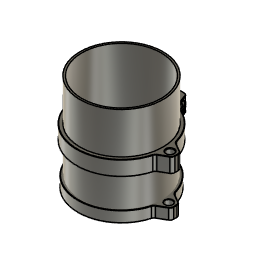
rear_44mm_dia (Autodesk Fusion 360 design; units mm, degrees)
Autodesk Fusion 360 part; units mm, degrees
sketch "Sketch1" plane through (0, 0, 0) normal (0, 0, 1) x (1, 0, 0)
  circle A0 centre (0, 0) radius 22.2
  circle A1 centre (0, 0) radius 21.2
  dimension "d1" = 44.4
  dimension "d2" = 1
  constraint coincident A0.centre A1.centre
  measures "d1" diameter of A0
  measures "d2" distance of A0 A1
extrude "Extrude1" add sketch "Sketch1" along normal blind 50 makes body 1
ref_plane "WorkPlane1" through (0, 0, 20) normal (0, 0, 1) x (1, 0, 0)
sketch "Sketch2" plane through (0, 0, 20) normal (0, 0, 1) x (1, 0, 0)
  circle A0 centre (0, 0) radius 22
  circle A1 centre (0, 0) radius 24
  line L0 (0, 0) -> (0, 24) construction
  line L1 (-6.9118, 22.9832) -> (-4, 30.9832)
  line L2 (-4, 30.9832) -> (0, 30.9832)
  line L3 (0, 30.9832) -> (0, 24)
  line L4 (-6.9118, 22.9832) -> (0, 22.9832) construction
  line L5 (-4, 30.9832) -> (-4, 22.9832) construction
  line L6 (0, 0) -> (-0.3072, 21.9979)
  line L7 (-0.3072, 21.9979) -> (-0.3072, 30.9832)
  line L8 (6.9118, 22.9832) -> (4, 30.9832)
  line L9 (4, 30.9832) -> (0, 30.9832)
  line L10 (0.3072, 21.9979) -> (0.3072, 30.9832)
  line L11 (0, 0) -> (0.3072, 21.9979)
  circle A2 centre (-26, 0) radius 2
  line L12 (0, 0) -> (-24, 0) construction
  line L13 (-23.3435, 5.5752) -> (-29.5, 2.0207)
  line L14 (-29.5, 2.0207) -> (-29.5, 0)
  line L15 (-23.3435, -5.5752) -> (-29.5, -2.0207)
  line L16 (-29.5, -2.0207) -> (-29.5, 0)
  line L17 (23.3435, 5.5752) -> (29.5, 2.0207)
  line L18 (29.5, 2.0207) -> (29.5, 0)
  line L19 (29.5, -2.0207) -> (29.5, 0)
  line L20 (23.3435, -5.5752) -> (29.5, -2.0207)
  circle A3 centre (26, 0) radius 2
  dimension "d6" = 44
  dimension "d7" = 2
  dimension "d8" = 8
  dimension "d9" = 20
  dimension "d10" = 4
  dimension "d11" = 0.8
  dimension "d14" = 4
  dimension "d16" = 3.5
  dimension "d17" = 3.5
  dimension "d18" = 120
  constraint coincident A0.centre A1.centre
  constraint coincident A1 L0.end
  constraint vertical L0
  constraint coincident A1 L1.start
  constraint horizontal L2
  constraint perpendicular L2 L3
  constraint coincident L0 L4.end
  constraint horizontal L4
  constraint coincident L4 L5.end
  constraint perpendicular L4 L5
  constraint coincident A0 L6.end
  constraint coincident L2 L7.end
  constraint perpendicular L2 L7
  constraint symmetric L0 L1.start L8.start
  constraint symmetric L0 L1.end L8.end
  constraint symmetric L0 L2.end L3.start
  constraint symmetric L0 A0.centre A1.centre
  constraint symmetric L0 L6.end L10.start
  constraint symmetric L0 L7.end L10.end
  constraint coincident A1 L12.end
  constraint horizontal L12
  constraint coincident A2.centre L12
  constraint coincident A1 L13.start
  constraint vertical L14
  constraint tangent A1 A2
  constraint coincident L12 L14.end
  constraint symmetric L12 L13.start L15.start
  constraint symmetric L12 L13.end L15.end
  constraint symmetric L12 L14.end L16.end
  constraint symmetric L0 A2 A3
  constraint symmetric L0 L13.start L17.start
  constraint symmetric L0 L13.end L17.end
  constraint symmetric L0 L14.end L18.end
  constraint symmetric L0 L15.start L20.start
  constraint symmetric L0 L15.end L19.start
  measures "d6" diameter of A0
  measures "d7" distance of A0 A1
  measures "d8" distance of L2 L4
  measures "d9" angle of L1 L5
  measures "d10" distance of L1.end L3
  measures "d11" angle of L0 L6
  measures "d14" diameter of A2
  measures "d16" distance of A2.centre L14
  measures "d17" distance of A2.centre L13
  measures "d18" angle of L13 L14
extrude "Extrude2" add sketch "Sketch2" along normal blind 8 separate body contours A0 A1 L7 L10 | A1 L8 L9 L10 | A1 L1 L2 L7 | A1 L17 L18 L19 L20 | A1 L13 L14 L15 L16 picked at (22.5633, -1.6974) makes body 2
sketch "Sketch3" plane through (-0.3072, 0, 0) normal (1, 0, 0) x (0, 1, 0)
  line L0 (21.9979, 20) -> (30.9832, 20)
  line L1 (30.9832, 20) -> (30.9832, 28)
  line L2 (30.9832, 28) -> (21.9979, 28)
  line L3 (21.9979, 28) -> (21.9979, 20)
  line L4 (21.9979, 24) -> (30.9832, 24) construction
  line L5 (26.4905, 28) -> (26.4905, 20) construction
  circle A0 centre (26.9832, 24) radius 1.4
  dimension "d19" = 2.8
  dimension "d20" = 4
  constraint midpoint L3 L4.start
  constraint midpoint L1 L4.end
  constraint midpoint L2 L5.start
  constraint perpendicular L2 L5
  constraint coincident L4 A0.centre
  measures "d19" diameter of A0
  measures "d20" distance of L1 A0.centre
extrude "Extrude3" cut sketch "Sketch3" along normal through all and the other way through all contours A0 bodies 2
sketch "Sketch4" plane through (0, 0, 28) normal (0, 0, 1) x (-1, 0, 0)
  circle A0 centre (-26, 0) radius 2
  circle A1 centre (26, 0) radius 2
  arc A2 (23.3435, 5.5752) -> (-23.3435, 5.5752) centre (0, 0) ccw
  line L0 (-23.3435, 5.5752) -> (-29.5, 2.0207)
  line L1 (-29.5, 2.0207) -> (-29.5, -2.0207)
  line L2 (-29.5, -2.0207) -> (-23.3435, -5.5752)
  arc A3 (-23.3435, -5.5752) -> (-6.9118, -22.9832) centre (0, 0) ccw
  line L3 (-6.9118, -22.9832) -> (-4, -30.9832)
  line L4 (-4, -30.9832) -> (-0.3072, -30.9832)
  line L5 (-0.3072, -30.9832) -> (-0.3072, -21.9979)
  arc A4 (0.3072, -21.9979) -> (-0.3072, -21.9979) centre (0, 0) ccw
  line L6 (0.3072, -21.9979) -> (0.3072, -30.9832)
  line L7 (0.3072, -30.9832) -> (4, -30.9832)
  line L8 (4, -30.9832) -> (6.9118, -22.9832)
  arc A5 (6.9118, -22.9832) -> (23.3435, -5.5752) centre (0, 0) ccw
  line L9 (23.3435, -5.5752) -> (29.5, -2.0207)
  line L10 (29.5, -2.0207) -> (29.5, 2.0207)
  line L11 (29.5, 2.0207) -> (23.3435, 5.5752)
  line L12 (-4, -30.9832) -> (-4, -21.6333) construction
  constraint coincident L3.end L4.start
  constraint coincident A4 L12.end
  constraint perpendicular L4 L12
sketch "Sketch5" plane through (0, 0, 20) normal (0, 0, -1) x (1, 0, 0)
  circle A0 centre (26, 0) radius 2
  circle A1 centre (-26, 0) radius 2
  arc A2 (23.3435, 5.5752) -> (-23.3435, 5.5752) centre (0, 0) ccw
  line L0 (-23.3435, 5.5752) -> (-29.5, 2.0207)
  line L1 (-29.5, 2.0207) -> (-29.5, -2.0207)
  line L2 (-29.5, -2.0207) -> (-23.3435, -5.5752)
  arc A3 (-23.3435, -5.5752) -> (-6.9118, -22.9832) centre (0, 0) ccw
  line L3 (-6.9118, -22.9832) -> (-4, -30.9832)
  line L4 (-4, -30.9832) -> (-0.3072, -30.9832)
  line L5 (-0.3072, -30.9832) -> (-0.3072, -21.9979)
  arc A4 (0.3072, -21.9979) -> (-0.3072, -21.9979) centre (0, 0) ccw
  line L6 (0.3072, -21.9979) -> (0.3072, -30.9832)
  line L7 (0.3072, -30.9832) -> (4, -30.9832)
  line L8 (4, -30.9832) -> (6.9118, -22.9832)
  arc A5 (6.9118, -22.9832) -> (23.3435, -5.5752) centre (0, 0) ccw
  line L9 (23.3435, -5.5752) -> (29.5, -2.0207)
  line L10 (29.5, -2.0207) -> (29.5, 2.0207)
  line L11 (29.5, 2.0207) -> (23.3435, 5.5752)
  line L12 (4, -30.9832) -> (4, -21.6333) construction
ref_plane "WorkPlane2" through (4, 30.9832, 28) normal (-1, 0, 0) x (0, -1, 0)
sketch "Sketch6" plane through (4, 0, 0) normal (-1, 0, 0) x (0, -1, 0)
  circle A0 centre (-26.9832, 24) radius 1.4
  circle A1 centre (-26.9832, 24) radius 1.4
  circle A2 centre (-26.9832, 24) radius 3
  dimension "d23" = 6
  constraint concentric A0 A2
  measures "d23" diameter of A2
extrude "Extrude4" cut sketch "Sketch6" against normal through all bodies 2
sketch "Sketch7" plane through (0.3072, 0, 0) normal (-1, 0, 0) x (0, -1, 0)
  circle A0 centre (-26.9832, 24) radius 1.4
  line L0 (-30.9832, 20) -> (-21.9979, 20)
  line L1 (-21.9979, 20) -> (-21.9979, 28)
  line L2 (-21.9979, 28) -> (-30.9832, 28)
  line L3 (-30.9832, 28) -> (-30.9832, 20)
  circle A1 centre (-26.9832, 24) radius 1.7
  dimension "d28" = 3.4
  constraint concentric A0 A1
  measures "d28" diameter of A1
extrude "Extrude6" cut sketch "Sketch7" against normal up to surface (3.6928 mm away) contours A1 bodies 2
fillet "Fillet1" radius 2 12 edges at (-29.5, -2.0207, 24) (-23.3435, -5.5752, 24) (-29.5, 2.0207, 24) (-23.3435, 5.5752, 24) (23.3435, -5.5752, 24) (29.5, -2.0207, 24) (29.5, 2.0207, 24) (23.3435, 5.5752, 24) (6.9118, 22.9832, 24) (-6.9118, 22.9832, 24) (4, 30.9832, 24) (-4, 30.9832, 24) on bodies 2
fillet "Fillet2" radius 0.5 4 edges at (0.3072, 30.9832, 24) (-0.3072, 30.9832, 24) (0.3072, 21.9979, 24) (-0.3072, 21.9979, 24) on bodies 2
chamfer "Chamfer1" distance 0.2 angle 45 4 edges at (4, 28.5682, 23.3853) (0.3072, 28.5682, 24.6147) (-0.3072, 25.6779, 24.5063) (-5.9654, 25.5832, 24) on bodies 2
fillet "Fillet5" radius 0.2 3 edges at (4, 29.7802, 22.9152) (6.5478, 23.9832, 24) (4.3316, 29.9832, 24) on bodies 2
chamfer "Chamfer2" distance 0.2 angle 45 32 edges at (-23.4884, 5.6646, 28) (-17.4982, 16.4259, 28) (-7.0551, 23.1595, 28) (-5.5281, 26.7847, 28) (-3.7467, 30.6215, 28) (-1.7034, 30.9832, 28) (-0.4536, 30.8368, 28) (-0.3072, 26.4844, 28) (-0.4473, 22.1384, 28) (0, -22, 28) (0.4473, 22.1384, 28) (0.3072, 26.4844, 28) (0.4536, 30.8368, 28) (1.7034, 30.9832, 28) (3.7467, 30.6215, 28) (5.5281, 26.7847, 28) (7.0551, 23.1595, 28) (17.4982, 16.4259, 28) (23.4884, 5.6646, 28) (26.2856, 3.8765, 28) (29.2321, 1.866, 28) (29.5, 0, 28) (29.2321, -1.866, 28) (26.2856, -3.8765, 28) (23.4884, -5.6646, 28) (0, -24, 28) (-23.4884, -5.6646, 28) (-26.2856, -3.8765, 28) (-29.2321, -1.866, 28) (-29.5, 0, 28) (-29.2321, 1.866, 28) (-26.2856, 3.8765, 28) on bodies 2
chamfer "Chamfer3" distance 0.3 angle 45 35 edges at (-27.8647, 0.7232, 28) (24.1353, 0.7232, 28) (26.2856, 3.8765, 20) (29.2321, 1.866, 20) (29.5, 0, 20) (29.2321, -1.866, 20) (26.2856, -3.8765, 20) (23.4884, -5.6646, 20) (0, -24, 20) (-23.4884, -5.6646, 20) (-26.2856, -3.8765, 20) (-29.2321, -1.866, 20) (-29.5, 0, 20) (-29.2321, 1.866, 20) (-26.2856, 3.8765, 20) (-23.4884, 5.6646, 20) (-17.4982, 16.4259, 20) (-7.0551, 23.1595, 20) (-5.5281, 26.7847, 20) (-3.7467, 30.6215, 20) (-1.7034, 30.9832, 20) (-0.4536, 30.8368, 20) (-0.3072, 26.4844, 20) (-0.4473, 22.1384, 20) (0, -22, 20) (0.4473, 22.1384, 20) (0.3072, 26.4844, 20) (0.4536, 30.8368, 20) (1.7034, 30.9832, 20) (3.7467, 30.6215, 20) (5.5281, 26.7847, 20) (7.0551, 23.1595, 20) (17.4982, 16.4259, 20) (23.4884, 5.6646, 20) (24.1353, 0.7232, 20) on bodies 2
sketch "Sketch8" plane through (0, 0, 0) normal (0, 0, 1) x (1, 0, 0)
  circle A0 centre (0, 0) radius 21.3
  circle A1 centre (0, 0) radius 23.3
  line L0 (22.6198, 5.5889) -> (28.8, 2.0207)
  line L1 (28.8, 2.0207) -> (28.8, 0)
  line L2 (0, 0) -> (23.3, 0) construction
  line L3 (22.6198, -5.5889) -> (28.8, -2.0207)
  line L4 (28.8, -2.0207) -> (28.8, 0)
  line L5 (0, 0) -> (0, 21.3) construction
  line L6 (-22.6198, 5.5889) -> (-28.8, 2.0207)
  line L7 (-28.8, 2.0207) -> (-28.8, 0)
  line L8 (-28.8, -2.0207) -> (-28.8, 0)
  line L9 (-22.6198, -5.5889) -> (-28.8, -2.0207)
  circle A2 centre (25.3, 0) radius 2
  circle A3 centre (-25.3, 0) radius 2
  line L10 (0, 0) -> (-25.3, 0) construction
  dimension "d38" = 42.6
  dimension "d39" = 2
  dimension "d41" = 3.5
  dimension "d42" = 3.5
  dimension "d43" = 120
  dimension "d46" = 4
  dimension "d47" = 4
  constraint coincident A0.centre A1.centre
  constraint coincident A1 L0.start
  constraint vertical L1
  constraint coincident A1 L2.end
  constraint horizontal L2
  constraint symmetric L0.start L2 L3.start
  constraint symmetric L0.end L2 L3.end
  constraint symmetric L1.end L2 L4.end
  constraint coincident A0 L5.end
  constraint perpendicular L2 L5
  constraint symmetric L0.start L5 L6.start
  constraint symmetric L0.end L5 L6.end
  constraint symmetric L1.end L5 L7.end
  constraint symmetric L3.start L5 L9.start
  constraint symmetric L3.end L5 L8.start
  constraint tangent A1 A2
  constraint coincident L2 A2.centre
  constraint tangent A1 A3
  constraint coincident A3.centre L10.end
  constraint horizontal L10
  measures "d38" diameter of A0
  measures "d39" distance of A0 A1
  measures "d41" distance of L0 A2.centre
  measures "d42" distance of L1 A2.centre
  measures "d43" angle of L0 L1
  measures "d46" diameter of A2
  measures "d47" diameter of A3
extrude "Extrude7" add sketch "Sketch8" along normal blind 4 separate body makes body 3
extrude "Extrude8" add sketch "Sketch8" against normal blind 2 contours A0 | A1 | A1 L0 L1 L3 L4 | A1 L6 L7 L8 L9 bodies 3
fillet "Fillet3" radius 2 8 edges at (22.6198, -5.5889, 1) (28.8, -2.0207, 1) (28.8, 2.0207, 1) (22.6198, 5.5889, 1) (-22.6198, 5.5889, 1) (-28.8, 2.0207, 1) (-28.8, -2.0207, 1) (-22.6198, -5.5889, 1) on bodies 3
chamfer "Chamfer4" distance 0.2 angle 45 19 edges at (-28.5321, -1.866, 4) (-28.8, 0, 4) (-28.5321, 1.866, 4) (-25.5697, 3.8858, 4) (-22.7616, 5.6764, 4) (0, 23.3, 4) (22.7616, 5.6764, 4) (25.5697, 3.8858, 4) (28.5321, 1.866, 4) (28.8, 0, 4) (28.5321, -1.866, 4) (25.5697, -3.8858, 4) (22.7616, -5.6764, 4) (0, -23.3, 4) (-22.7616, -5.6764, 4) (-25.5697, -3.8858, 4) (-27.1647, 0.7232, 4) (-19.8586, 7.7024, 4) (23.4353, 0.7232, 4) on bodies 3
chamfer "Chamfer5" distance 0.3 angle 45 18 edges at (25.5697, -3.8858, -2) (22.7616, -5.6764, -2) (0, -23.3, -2) (-22.7616, -5.6764, -2) (-25.5697, -3.8858, -2) (-28.5321, -1.866, -2) (-28.8, 0, -2) (-28.5321, 1.866, -2) (-25.5697, 3.8858, -2) (-22.7616, 5.6764, -2) (0, 23.3, -2) (22.7616, 5.6764, -2) (25.5697, 3.8858, -2) (28.5321, 1.866, -2) (28.8, 0, -2) (28.5321, -1.866, -2) (-27.1647, -0.7232, -2) (23.4353, -0.7232, -2) on bodies 3
fillet "Fillet4" radius 0.2 1 edges at (-19.8586, 7.7024, 0) on bodies 3
equation "d11 = ( 1.6 / 2 ) * 1 deg"
named bodies: "mocked_scope_44mm", "scope_collar", "scope_cap"
